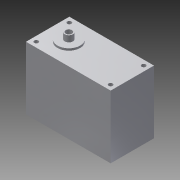
# Autodesk Inventor part: KRS-2542HV ICS
Saved by Autodesk Inventor 2015 (Build 190159000, 159)
## iProperties
Created: 2015-05-09
Part Number: KRS-2542HV ICS
Material: PVC、軟質
Document SubType Name: Modeling
Designer: kenta
Density: 1.3 g/cm^3
Appearance: PVC - 白
Mass: 35.558 g
Surface Area: 69.1615 cm^2
Volume: 25.655 cm^3
Author: kenta
Autodesk Inventor part; units mm, degrees
ref_plane "YZ Plane" through (0, 0, 0) normal (1, 0, 0) x (0, 1, 0)
ref_plane "XZ Plane" through (0, 0, 0) normal (0, 1, 0) x (-1, 0, 0)
ref_plane "XY Plane" through (0, 0, 0) normal (0, 0, 1) x (1, 0, 0)
sketch "スケッチ1" plane through (0, 0, 0) normal (0, 0, 1) x (1, 0, 0)
  line L0 (0, 0) -> (41, 0)
  line L1 (41, 0) -> (41, -21)
  line L2 (41, -21) -> (0, -21)
  line L3 (0, -21) -> (0, 0)
  dimension "d0" = 41
  dimension "d1" = 21
  constraints: 8 end point, 2 parallel, 1 horizontal, 1 perpendicular
  measures "d0" distance of L1.end L2.end
  measures "d1" distance of L0.end L1.end
extrude "押し出し1" add sketch "スケッチ1" along normal blind 30.5
sketch "スケッチ2" plane through (0, 0, 0) normal (0, 0, -1) x (-1, 0, 0)
  line L0 (0, 0) -> (-41, 0) projected
  line L1 (0, -21) -> (0, 0) projected
  line L2 (-41, 0) -> (-41, -21) projected
  line L3 (0, -21) -> (-41, -21) projected
  point P0 (-2.5, -2.5)
  point P1 (-38.5, -2.5)
  point P2 (-2.5, -18.5)
  point P3 (-38.5, -18.5)
  dimension "d32" = 16
  dimension "d33" = 2.5
  dimension "d34" = 36
  dimension "d35" = 2.5
  dimension "d36" = 2.5
  dimension "d37" = 36
  dimension "d39" = 16
  dimension "d40" = 2.5
  constraints: 1 horizontal alignment
  measures "d32" distance of point (-2.5, -2.5) point (-2.5, -18.5)
  measures "d33" distance from line of point (-2.5, -2.5) L0
  measures "d34" distance of point (-38.5, -2.5) point (-2.5, -2.5)
  measures "d35" distance from line of point (-2.5, -2.5) L1
  measures "d36" distance from line of point (-2.5, -18.5) L1
  measures "d37" distance of point (-38.5, -18.5) point (-2.5, -18.5)
  measures "d39" distance of point (-38.5, -2.5) point (-38.5, -18.5)
  measures "d40" distance from line of point (-2.5, -18.5) L3
hole "穴1" at (2.5, -2.5, 0) at (38.5, -2.5, 0) at (2.5, -18.5, 0) at (38.5, -18.5, 0) direction (0, 0, 1) diameter 2 end through all
sketch "スケッチ3" plane through (0, 0, 0) normal (0, 0, -1) x (-1, 0, 0)
  circle A0 centre (-10.25, -10.5) radius 5.5
  point P0 (0, 0)
  dimension "d11" = 11
  constraints: 1 centre point, 1 coincident
  measures "d11" diameter of A0
extrude "押し出し2" add sketch "スケッチ3" along normal blind 1
sketch "スケッチ4" plane through (10.25, -10.5, -1) normal (0, 0, -1) x (-1, 0, 0)
  circle A0 centre (0, 0) radius 1.5
  point P0 (10.25, 10.5)
  dimension "d14" = 3
  constraints: 1 centre point
  measures "d14" diameter of A0
extrude "押し出し3" cut sketch "スケッチ4" against normal blind 40
sketch "スケッチ5" plane through (10.25, -10.5, -1) normal (0, 0, -1) x (-1, 0, 0)
  circle A0 centre (0, 0) radius 2
  point P0 (10.25, 10.5)
  dimension "d17" = 4
  constraints: 1 centre point
  measures "d17" diameter of A0
extrude "押し出し4" add sketch "スケッチ5" along normal blind 3
sketch "スケッチ6" plane through (10.25, -10.5, -4) normal (0, 0, -1) x (-1, 0, 0)
  circle A0 centre (0, 0) radius 1.5
  point P0 (10.25, 10.5)
  dimension "d20" = 3
  constraints: 1 centre point
  measures "d20" diameter of A0
extrude "押し出し5" cut sketch "スケッチ6" against normal blind 4
sketch "スケッチ8" plane through (0, 0, 30.5) normal (0, 0, 1) x (1, 0, 0)
  circle A0 centre (10.25, -10.5) radius 5.5
  point P0 (0, 0)
  dimension "d23" = 11
  constraints: 1 centre point
  measures "d23" diameter of A0
extrude "押し出し6" add sketch "スケッチ8" along normal blind 1
sketch "スケッチ9" plane through (10.25, -10.5, 31.5) normal (0, 0, 1) x (1, 0, 0)
  circle A0 centre (0, 0) radius 1.5 projected
  circle A1 centre (0, 0) radius 2
  point P0 (-10.25, 10.5)
  dimension "d26" = 4
  constraints: 1 centre point, 1 coincident
  measures "d26" diameter of A1
extrude "押し出し7" add sketch "スケッチ9" along normal blind 3
sketch "スケッチ10" plane through (10.25, -10.5, 31.5) normal (0, 0, 1) x (1, 0, 0)
  circle A0 centre (0, 0) radius 1.5
  point P0 (-10.25, 10.5)
  dimension "d29" = 3
  constraints: 1 centre point
  measures "d29" diameter of A0
extrude "押し出し8" cut sketch "スケッチ10" against normal blind 3
